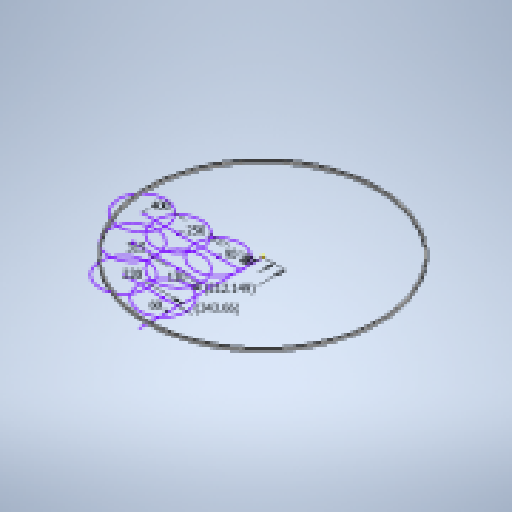
# Autodesk Inventor part: PRS 940-512 DIM filter-distribution-system 1000
Saved by Autodesk Inventor 2025.1 (Build 291241020, 241B)
## iProperties
Created: 2025-06-24
Part Number: PRS 940-512 DIM filter-distribution-system 1000
Material: Generic
Document SubType Name: Modeling
Designer: admin
Density: 1 g/cm^3
Sheet Metal Rule: Default
Appearance: Default
way_tube_L5: 120.000 mm
way_tube_L6: 90.000 mm
way_tube_L7: 20.000 mm
way_tube_L8: 90.000 mm
way_tube_L9: 80.000 mm
way_tube_L10: 80.000 mm
Author: user
Autodesk Inventor part; units mm, degrees
ref_plane "YZ Plane" through (0, 0, 0) normal (1, 0, 0) x (0, 1, 0)
ref_plane "XZ Plane" through (0, 0, 0) normal (0, 1, 0) x (-1, 0, 0)
ref_plane "XY Plane" through (0, 0, 0) normal (0, 0, 1) x (1, 0, 0)
sketch "Sketch1" plane through (0, 0, 0) normal (0, 0, 1) x (1, 0, 0)
  circle A0 centre (0, 0) radius 470
  circle A1 centre (0, 0) radius 464
  dimension "d0" = 940
  dimension "d1" = 6
  constraints: 2 centre point, 1 coincident
  measures "d0" diameter of A0
  measures "d1" radial gap between concentric circles of A0 A1
extrude "Extrusion1" add sketch "Sketch1" along normal blind 10
sketch "Sketch2" plane through (0, 0, 0) normal (0, 0, 1) x (1, 0, 0)
  circle A0 centre (-90, -87.958) radius 95
  circle A1 centre (-250, -87.958) radius 95
  circle A2 centre (-398.347, -87.958) radius 95
  circle A3 centre (-128.347, -210) radius 95
  circle A4 centre (-313.347, -210) radius 95
  circle A5 centre (-218.347, -340) radius 95
  line L0 (1.653, -87.958) -> (-398.347, -87.958)
  line L1 (1.653, 2.1491) -> (1.653, -497.8509)
  line L2 (1.653, -340) -> (-218.347, -340)
  line L3 (1.653, -210) -> (-313.347, -210)
  circle A6 centre (-88.347, -340) radius 95
  point P0 (0, 0)
  dimension "d8" = 210
  dimension "d9" = 340
  dimension "d11" = 90
  dimension "d12" = 250
  dimension "d13" = 400
  dimension "d16" = 130
  dimension "d17" = 315
  dimension "d18" = 90
  dimension "d19" = 220
  constraints: 8 end point, 7 centre point, 7 point on line, 3 perpendicular, 1 coincident, 1 horizontal
  measures "d8" distance from line of L3 point (0, 0)
  measures "d9" distance from line of point (0, 0) L2
  measures "d11" horizontal distance of A0.centre point (0, 0)
  measures "d12" horizontal distance of A1.centre point (0, 0)
  measures "d13" distance from line of L0.end L1
  measures "d16" distance from line of L1 A3.centre
  measures "d17" distance from line of L1 A4.centre
  measures "d18" distance from line of A6.centre L1
  measures "d19" distance of L2.start L2.end
sketch "Sketch3" plane through (0, 0, 0) normal (0, 0, 1) x (1, 0, 0)
  circle A0 centre (-104.0992, -233.3488) radius 95
  circle A1 centre (-161.9131, -395.3117) radius 95
  circle A2 centre (-91.7953, -514.3257) radius 95
  circle A3 centre (-280.9346, -260.412) radius 95
  circle A4 centre (-299.5406, -418.8761) radius 95
  circle A5 centre (-250.7395, 99.5106) radius 95
  circle A6 centre (-395.8303, 87.9315) radius 95
  circle A7 centre (-535.2648, 91.0733) radius 95
  circle A8 centre (-460.3613, -287.8718) radius 95
  circle A9 centre (-531.2922, -111.9436) radius 95
  circle A10 centre (-392.3143, -102.4845) radius 95
  circle A11 centre (0, 0) radius 542.9574 construction
  circle A12 centre (-253.2201, -93.0176) radius 95
  circle A13 centre (-90.4998, -81.9426) radius 95
  circle A14 centre (85.6841, -88.1302) radius 95
  circle A15 centre (-90.4998, 88.0537) radius 95
  circle A16 centre (0, 0) radius 405.4794 construction
  circle A17 centre (0, 0) radius 269.7641 construction
  circle A18 centre (85.6841, 88.0537) radius 95
  line L0 (0, 0) -> (0, -542.9574)
  line L1 (0, -75.783) -> (-531.2922, -111.9436)
  line L2 (0, -217.4173) -> (-460.3613, -287.8718)
  circle A19 centre (0, 0) radius 600
  line L3 (0, -367.5891) -> (-299.5406, -418.8761)
  line L4 (-91.7953, -514.3257) -> (0, -514.3257)
  point P0 (0, 0)
  dimension "d21" = 190
  dimension "d22" = 1200
  constraints: 20 centre point, 15 equal radius, 10 end point, 10 point on line, 8 point on circle, 5 coincident, 1 perpendicular, 1 vertical
  measures "d21" diameter of A14
  measures "d22" diameter of A19
equation "\"GapSize\" = Thickness"
equation "\"BendRadius\" = Thickness"
equation "\"MinimumRemnant\" = 2 * Thickness"
equation "\"BendReliefDepth\" = 0.5 * Thickness"
equation "\"BendReliefWidth\" = Thickness"
equation "\"CornerReliefSize\" = 4 * Thickness"
equation "\"JacobiRadiusSize\" = BendRadius"
equation "\"TransitionRadius\" = BendRadius"
equation "\"way_tube_L1\" = 1"
equation "\"way_tube_L2\" = 1"
equation "\"way_tube_L3\" = 1"
equation "\"way_tube_L4\" = 1"
equation "\"way_tube_L5\" = 120"
equation "\"way_tube_L6\" = 90"
equation "\"way_tube_L7\" = 20"
equation "\"way_tube_L8\" = 90"
equation "\"way_tube_L9\" = 80"
equation "\"way_tube_L10\" = 80"
equation "\"Thickness\" = 3.048"
body "Solid1"
